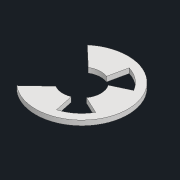
# Autodesk Inventor part: 7mm E-Clip
Saved by Autodesk Inventor 2022 (Build 260153000, 153)
## iProperties
Created: 2022-09-24
Part Number: 7mm E-Clip
Material: Generic
Document SubType Name: Modeling
Designer: robpl
Density: 1 g/cm^3
Appearance: Iron Gray
Author: robpl
Autodesk Inventor part; units mm, degrees
ref_plane "YZ Plane" through (0, 0, 0) normal (1, 0, 0) x (0, 1, 0)
ref_plane "XZ Plane" through (0, 0, 0) normal (0, 1, 0) x (-1, 0, 0)
ref_plane "XY Plane" through (0, 0, 0) normal (0, 0, 1) x (1, 0, 0)
sketch "Sketch1" plane through (0, 0, 0) normal (0, 1, 0) x (-1, 0, 0)
  circle A0 centre (0, 0) radius 8.5
  circle A1 centre (0, 0) radius 3.5
  circle A2 centre (0, 0) radius 7
  line L0 (5.4772, 6.5) -> (1.8028, 3)
  line L1 (1.8028, -3) -> (5.4772, -6.5)
  line L2 (-1.299, 3.25) -> (-2.0392, 6.6964)
  line L3 (-2.8723, 2) -> (-6.0622, 3.5)
  line L4 (-2.8723, -2) -> (-6.0622, -3.5)
  line L5 (-1.299, -3.25) -> (-2.0392, -6.6964)
  dimension "d0" = 17
  dimension "d2" = 6
  dimension "d3" = 14
  dimension "d4" = 13
  dimension "d5" = 4
  dimension "d6" = 7
  dimension "d8" = 7
  dimension "d9" = 6.5
  constraints: 12 end point, 12 point on circle, 5 vertical alignment, 4 coincident, 4 equal length, 3 centre point
  measures "d0" diameter of A0
  measures "d2" distance of L1.start L0.end
  measures "d3" diameter of A2
  measures "d4" distance of L1.end L0.start
  measures "d5" distance of L3.start L4.start
  measures "d6" distance of L4.end L3.end
  measures "d8" diameter of A1
  measures "d9" distance of L2.start L5.start
extrude "Extrusion1" add sketch "Sketch1" along normal blind 0.9 contours L0 A2 L1 A0 | L0 A1 L2 A2 | A2 L5 A1 L1 | L3 A1 L4 A2 picked at (-7.9468, 0.2439)
body "Solid1"
